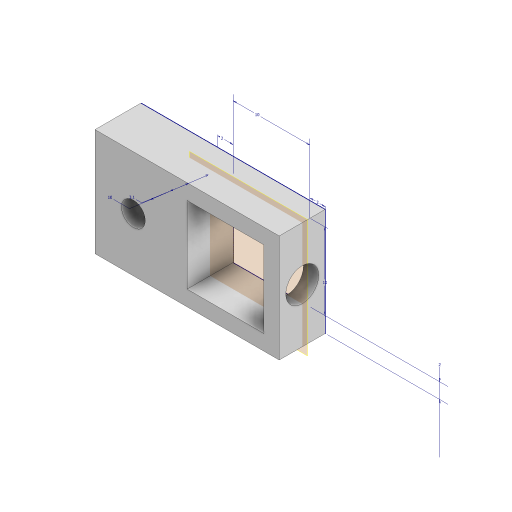
# Autodesk Inventor part: magnetic_holder_0217
Saved by Autodesk Inventor 2024 (Build 280153000, 153)
## iProperties
Created: 2023-02-16
Part Number: magnetic_holder_0217
Material: 一般
Document SubType Name: Modeling
Designer: USER
Density: 1 g/cm^3
Appearance: 預設
Author: USER
Autodesk Inventor part; units mm, degrees
ref_plane "YZ Plane" through (0, 0, 0) normal (1, 0, 0) x (0, 1, 0)
ref_plane "XZ Plane" through (0, 0, 0) normal (0, 1, 0) x (-1, 0, 0)
ref_plane "XY Plane" through (0, 0, 0) normal (0, 0, 1) x (1, 0, 0)
sketch "草圖1" plane through (0, 0, 0) normal (0, 0, 1) x (1, 0, 0)
  line L0 (0, 0) -> (14, 0)
  line L1 (14, 0) -> (14, 14)
  line L2 (14, 14) -> (0, 14)
  line L3 (0, 14) -> (0, 0)
  line L4 (12, 12) -> (2, 12)
  line L5 (2, 12) -> (2, 2)
  line L6 (2, 2) -> (12, 2)
  line L7 (12, 2) -> (12, 12)
  line L8 (2, 7) -> (12, 7) construction
  line L9 (0, 7) -> (14, 7) construction
  line L10 (0, 14) -> (-10, 14)
  line L11 (-10, 14) -> (-10, 0)
  line L12 (-10, 0) -> (0, 0)
  line L13 (0, 0) -> (0, 14)
  circle A0 centre (-5, 7) radius 1.55
  line L14 (2, 0) -> (2, 14)
  circle A1 centre (-5, 7) radius 5 construction
  point P0 (2, 2)
  dimension "d5" = 10
  dimension "d6" = 10
  dimension "d9" = 2
  dimension "d25" = 2
  dimension "d30" = 2
  dimension "d41" = 3.1
  dimension "d51" = 10
  constraints: 30 end point, 6 parallel, 4 midpoint, 4 perpendicular, 3 horizontal, 3 point on line, 2 centre point, 2 collinear, 2 tangent, 1 coincident
  measures "d5" distance of L4.start L4.end
  measures "d6" distance of L6.end L4.start
  measures "d9" distance between parallel lines of L7 L1
  measures "d25" distance between parallel lines of L0 L6
  measures "d30" distance between parallel lines of L3 L5
  measures "d41" diameter of A0
  measures "d51" diameter of A1
extrude "擠出1" add sketch "草圖1" along normal blind 6 contours L3 L2 L14 L5 L0 | L14 L6 L7 L4 L2 L1 L0
sketch "草圖5" plane through (14, 0, 0) normal (1, 0, 0) x (0, 0, -1)
  line L0 (0, 0) -> (0, 14) projected
  line L1 (0, 14) -> (-6, 14) projected
  line L2 (-6, 0) -> (-6, 14) projected
  line L3 (0, 0) -> (-6, 0) projected
  line L4 (0, 0) -> (0, 14) construction
  line L5 (0, 7) -> (-6, 7) construction
  line L6 (-6, 0) -> (-6, 14) construction
  line L7 (0, 14) -> (-6, 14) construction
  line L8 (-3, 14) -> (-3, 0) construction
  line L9 (0, 0) -> (-6, 0) construction
  circle A0 centre (-3, 7) radius 2.15
  dimension "d26" = 4.3
  constraints: 5 midpoint, 4 end point, 1 centre point
  measures "d26" diameter of A0
extrude "擠出5" cut sketch "草圖5" against normal blind 2 contours A0
ref_plane "工作平面2" through (0, 0, 3) normal (0, 0, 1) x (1, 0, 0)
extrude "擠出12" add sketch "草圖1" along normal mid plane 6 from surface at 3 contours L12 L11 L10 L3
